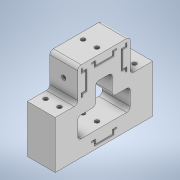
# Autodesk Inventor part: din_damper_connector
Saved by Autodesk Inventor 2021 (Build 250183000, 183)
## iProperties
Created: 2020-10-27
Part Number: din_damper_connector
Material: Generic
Document SubType Name: Modeling
Designer: Mateusz
Density: 1 g/cm^3
Appearance: Default
Author: Mateusz
Autodesk Inventor part; units mm, degrees
ref_plane "YZ Plane" through (0, 0, 0) normal (1, 0, 0) x (0, 1, 0)
ref_plane "XZ Plane" through (0, 0, 0) normal (0, 1, 0) x (-1, 0, 0)
ref_plane "XY Plane" through (0, 0, 0) normal (0, 0, 1) x (1, 0, 0)
sketch "Sketch1" plane through (0, 0, 0) normal (0, 1, 0) x (-1, 0, 0)
  line L0 (0, 0) -> (0, -140)
  line L1 (0, -140) -> (40, -140)
  line L2 (40, -140) -> (40, 0)
  line L3 (40, 0) -> (0, 0)
  dimension "d0" = 140
  dimension "d1" = 40
  constraints: 8 end point, 2 perpendicular, 1 horizontal, 1 vertical
  measures "d0" distance of L0.start L0.end
  measures "d1" distance of L0.end L1.end
extrude "Extrusion1" add sketch "Sketch1" along normal blind 68.5
sketch "Sketch2" plane through (0, 0, 0) normal (1, 0, 0) x (0, 0, -1)
  line L0 (140, 68.5) -> (0, 68.5) projected
  line L1 (45, 78.5) -> (39, 78.5)
  line L2 (39, 78.5) -> (39, 74.5)
  line L3 (39, 74.5) -> (37.3, 74.5)
  line L4 (37.3, 74.5) -> (37.3, 80.2)
  line L5 (37.3, 80.2) -> (43.5, 80.2)
  line L6 (43.5, 80.2) -> (43.5, 104.7)
  line L7 (43.5, 104.7) -> (37.3, 104.7)
  line L8 (37.3, 104.7) -> (37.3, 110.4)
  line L9 (37.3, 110.4) -> (39, 110.4)
  line L10 (39, 110.4) -> (39, 106.4)
  line L11 (39, 106.4) -> (45, 106.4)
  line L12 (45, 106.4) -> (45, 78.5)
  line L13 (95, 78.5) -> (101, 78.5)
  line L14 (101, 78.5) -> (101, 74.5)
  line L15 (101, 74.5) -> (102.7, 74.5)
  line L16 (102.7, 74.5) -> (102.7, 80.2)
  line L17 (102.7, 80.2) -> (96.5, 80.2)
  line L18 (96.5, 80.2) -> (96.5, 104.7)
  line L19 (96.5, 104.7) -> (102.7, 104.7)
  line L20 (102.7, 104.7) -> (102.7, 110.4)
  line L21 (102.7, 110.4) -> (101, 110.4)
  line L22 (101, 110.4) -> (101, 106.4)
  line L23 (101, 106.4) -> (95, 106.4)
  line L24 (95, 106.4) -> (95, 78.5)
  line L25 (37.3, 68.5) -> (32.3, 68.5)
  line L26 (32.3, 68.5) -> (32.3, 110.4)
  line L27 (32.3, 110.4) -> (32.3, 115.4)
  line L28 (32.3, 115.4) -> (102.7, 115.4)
  line L29 (102.7, 115.4) -> (107.7, 115.4)
  line L30 (107.7, 115.4) -> (107.7, 68.5)
  line L31 (37.3, 68.5) -> (107.7, 68.5)
  point P0 (0, 0)
  dimension "d8" = 4
  dimension "d9" = 1.7
  dimension "d10" = 5.7
  dimension "d11" = 6.2
  dimension "d12" = 24.5
  dimension "d13" = 5.7
  dimension "d14" = 1.7
  dimension "d15" = 4
  dimension "d16" = 6
  dimension "d17" = 5
  dimension "d18" = 5
  dimension "d19" = 5
  constraints: 62 end point, 8 perpendicular, 5 point on line, 4 horizontal, 3 vertical, 1 collinear
  measures "d8" distance of L1.end L2.end
  measures "d9" distance of L2.end L3.end
  measures "d10" distance of L3.end L4.end
  measures "d11" distance of L4.end L5.end
  measures "d12" distance of L5.end L6.end
  measures "d13" distance of L7.end L8.end
  measures "d14" distance of L8.end L9.end
  measures "d15" distance of L9.end L10.end
  measures "d16" distance of L10.end L11.end
  measures "d17" distance of L25.start L25.end
  measures "d18" distance of L26.end L27.end
  measures "d19" distance of L28.end L29.end
extrude "Extrusion2" add sketch "Sketch2" against normal up to surface (40 mm away)
sketch "Sketch3" plane through (0, 0, 0) normal (1, 0, 0) x (0, 0, -1)
  line L0 (87.95, 12.7) -> (87.95, 11)
  line L1 (87.95, 11) -> (83.95, 11)
  line L2 (83.95, 11) -> (83.95, 5)
  line L3 (83.95, 5) -> (70, 5)
  line L4 (70, 6.5) -> (82.25, 6.5)
  line L5 (82.25, 6.5) -> (82.25, 12.7)
  line L6 (82.25, 12.7) -> (87.95, 12.7)
  line L7 (52.05, 12.7) -> (52.05, 11)
  line L8 (52.05, 11) -> (56.05, 11)
  line L9 (56.05, 11) -> (56.05, 5)
  line L10 (56.05, 5) -> (70, 5)
  line L11 (70, 6.5) -> (57.75, 6.5)
  line L12 (57.75, 6.5) -> (57.75, 12.7)
  line L13 (57.75, 12.7) -> (52.05, 12.7)
  line L14 (107.7, 115.4) -> (32.3, 115.4) projected
  line L15 (87.95, 110.4) -> (87.95, 108.7)
  line L16 (87.95, 108.7) -> (83.95, 108.7)
  line L17 (83.95, 108.7) -> (83.95, 102.7)
  line L18 (83.95, 102.7) -> (70, 102.7)
  line L19 (70, 104.2) -> (82.25, 104.2)
  line L20 (82.25, 110.4) -> (87.95, 110.4)
  line L21 (52.05, 110.4) -> (52.05, 108.7)
  line L22 (52.05, 108.7) -> (56.05, 108.7)
  line L23 (56.05, 108.7) -> (56.05, 102.7)
  line L24 (56.05, 102.7) -> (70, 102.7)
  line L25 (70, 104.2) -> (57.75, 104.2)
  line L26 (57.75, 104.2) -> (57.75, 110.4)
  line L27 (57.75, 110.4) -> (52.05, 110.4)
  line L28 (82.25, 104.2) -> (82.25, 110.4)
  line L29 (140, 0) -> (0, 0) projected
  dimension "d27" = 6
  dimension "d31" = 6
  constraints: 56 end point, 4 perpendicular
  measures "d27" distance of L1.end L2.end
  measures "d31" distance of L17.start L17.end
extrude "Extrusion3" cut sketch "Sketch3" against normal up to surface (40 mm away)
sketch "Sketch4" plane through (0, 115.4, -32.3) normal (0, 1, 0) x (1, 0, 0)
  line L0 (-40, 75.4) -> (-40, 0) projected
  line L1 (0, 0) -> (-40, 0) projected
  line L2 (0, 75.4) -> (0, 0) projected
  line L3 (0, 75.4) -> (-40, 75.4) projected
  line L4 (0, -32.3) -> (0, 107.7) projected
  line L5 (-40, 107.7) -> (-40, -32.3) projected
  line L6 (-40, 75.4) -> (0, 75.4) projected
  line L7 (0, 0) -> (-40, 0) projected
  circle A0 centre (-30, 37.7) radius 3.05
  circle A1 centre (-10, 37.7) radius 3.05
  dimension "d48" = 6.1
  dimension "d49" = 6.1
  constraints: 2 centre point
  measures "d48" diameter of A0
  measures "d49" diameter of A1
sketch "Sketch5" plane through (0, 68.5, -107.7) normal (0, 0, -1) x (-1, 0, 0)
  line L0 (40, 0) -> (40, 46.9) projected
  line L1 (0, 46.9) -> (40, 46.9) projected
  line L2 (0, 0) -> (0, 46.9) projected
  line L3 (40, 0) -> (0, 0) projected
  line L4 (0, 46.9) -> (0, 0) projected
  line L5 (40, 36.2) -> (40, 11.7) projected
  line L6 (0, 46.9) -> (40, 46.9) projected
  circle A0 centre (20, 23.45) radius 3.05
  point P0 (0, -68.5)
  constraints: 1 centre point
sketch "Sketch6" plane through (0, 68.5, 0) normal (0, 1, 0) x (1, 0, 0)
  line L0 (-40, 107.7) -> (0, 107.7) projected
  line L1 (0, 107.7) -> (0, 140) projected
  line L2 (0, 140) -> (-40, 140) projected
  line L3 (-40, 140) -> (-40, 107.7) projected
  line L4 (0, 32.3) -> (-40, 32.3) projected
  line L5 (-40, 32.3) -> (-40, 0) projected
  line L6 (-40, 0) -> (0, 0) projected
  line L7 (0, 0) -> (0, 32.3) projected
  line L8 (0, 107.7) -> (0, 140) projected
  line L9 (-40, 140) -> (-40, 107.7) projected
  line L10 (0, 140) -> (-40, 140) projected
  line L11 (0, 32.3) -> (-40, 32.3) projected
  line L12 (-40, 0) -> (0, 0) projected
  line L13 (0, 0) -> (0, 140) projected
  line L14 (-40, 140) -> (-40, 0) projected
  circle A0 centre (-10, 123.85) radius 3.05
  circle A1 centre (-30, 123.85) radius 3.05
  circle A2 centre (-10, 16.15) radius 3.05
  circle A3 centre (-30, 16.15) radius 3.05
  dimension "d37" = 6.1
  dimension "d38" = 6.1
  dimension "d39" = 6.1
  dimension "d40" = 6.1
  constraints: 4 centre point
  measures "d37" diameter of A0
  measures "d38" diameter of A1
  measures "d39" diameter of A2
  measures "d40" diameter of A3
extrude "Extrusion4" cut sketch "Sketch6" against normal up to surface (68.5 mm away) contours A0 | A1 | A2 | A3
extrude "Extrusion5" cut sketch "Sketch4" against normal up to surface (115.4 mm away) contours A0 | A1
extrude "Extrusion6" cut sketch "Sketch5" against normal up to surface (75.4 mm away) contours A0
sketch "Sketch7" plane through (0, 0, 0) normal (1, 0, 0) x (0, 0, -1)
  line L0 (107.7, 53.5) -> (107.7, 23.5)
  line L1 (107.7, 23.5) -> (32.3, 23.5)
  line L2 (32.3, 23.5) -> (32.3, 53.5)
  line L3 (70, 23.5) -> (64, 23.5)
  line L4 (64, 23.5) -> (76, 23.5)
  line L5 (58, 53.5) -> (58, 93.5)
  line L6 (58, 93.5) -> (76, 93.5)
  line L7 (76, 93.5) -> (82, 93.5)
  line L8 (82, 93.5) -> (82, 53.5)
  line L9 (32.3, 53.5) -> (58, 53.5)
  line L10 (82, 53.5) -> (107.7, 53.5)
  line L11 (82, 93.5) -> (82, 83.5)
  line L12 (82, 83.5) -> (58, 83.5)
  point P0 (0, 0)
  dimension "d52" = 6
  dimension "d53" = 12
  dimension "d58" = 40
  dimension "d59" = 6
  dimension "d61" = 10
  constraints: 26 end point, 8 perpendicular, 5 point on line, 1 midpoint, 1 vertical
  measures "d52" distance of L3.start L3.end
  measures "d53" distance of L3.end L4.end
  measures "d58" distance of L5.start L5.end
  measures "d59" distance of L6.end L7.end
  measures "d61" distance of L7.end L11.end
extrude "Extrusion7" cut sketch "Sketch7" against normal up to surface (40 mm away) contours L0 L1 L2 L9 L5 L12 L8 L10
fillet "Fillet1" radius 5 8 edges at (-20, 53.5, -82) (-20, 53.5, -58) (-20, 53.5, -32.3) (-20, 23.5, -32.3) (-20, 23.5, -107.7) (-20, 53.5, -107.7) (-20, 83.5, -58) (-20, 83.5, -82)
fillet "Fillet2" radius 5 4 edges at (-20, 115.4, -32.3) (-20, 68.5, -32.3) (-20, 115.4, -107.7) (-20, 68.5, -107.7)
body "Solid1"
